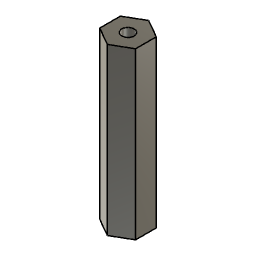
Drone_BodyStandoff v1 (Autodesk Fusion 360 design; units mm, degrees)
Autodesk Fusion 360 part; units mm, degrees
sketch "Sketch1" plane through (0, 0, 0) normal (0, 0, 1) x (1, 0, 0)
  line L0 (0, 5) -> (-4.3301, 2.5)
  line L1 (-4.3301, 2.5) -> (-4.3301, -2.5)
  line L2 (-4.3301, -2.5) -> (0, -5)
  line L3 (0, -5) -> (4.3301, -2.5)
  line L4 (4.3301, -2.5) -> (4.3301, 2.5)
  line L5 (4.3301, 2.5) -> (0, 5)
  dimension "d1" = 5
  measures "d1" distance of L0.start origin
extrude "Extrude1" add sketch "Sketch1" along normal blind 40
hole "Hole1" at (0, 0, 40) direction (0, 0, -1) diameter 4 depth 6 tip angle 118
hole "Hole2" at (0, 0, 0) direction (0, 0, 1) diameter 3 depth 6 tip angle 118
delete_face "DeleteFace1" 1 faces at (0.1991, -1.9901, 36)
hole "Hole3" at (0, 0, 40) direction (0, 0, -1) diameter 3 depth 6 tip angle 118
